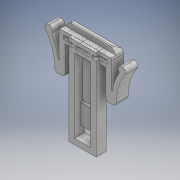
# Autodesk Inventor part: D5MG_Clip
Saved by Autodesk Inventor 2018 (Build 220112000, 112)
## iProperties
Created: 2017-08-14
Part Number: D5MG_Clip
Material: Типовые
Document SubType Name: Modeling
Designer: shawn
Density: 1 g/cm^3
Appearance: По умолчанию
Author: shawn
Autodesk Inventor part; units mm, degrees
ref_plane "YZ Plane" through (0, 0, 0) normal (1, 0, 0) x (0, 1, 0)
ref_plane "XZ Plane" through (0, 0, 0) normal (0, 1, 0) x (-1, 0, 0)
ref_plane "XY Plane" through (0, 0, 0) normal (0, 0, 1) x (1, 0, 0)
sketch "Эскиз1" plane through (0, 0, 0) normal (0, 1, 0) x (-1, 0, 0)
  line L0 (4.8, 15.9) -> (-4.8, 15.9)
  line L1 (-4.8, 15.9) -> (-4.8, -15.9)
  line L2 (-4.8, -15.9) -> (4.8, -15.9)
  line L3 (4.8, -15.9) -> (4.8, 15.9)
  line L4 (4.8, 15.9) -> (-4.8, -15.9) construction
  line L5 (-4.8, 15.9) -> (4.8, -15.9) construction
  line L6 (2.8, -13.9) -> (-2.8, -13.9)
  line L7 (-2.8, -13.9) -> (-2.8, 12.1)
  line L8 (-2.8, 12.1) -> (2.8, 12.1)
  line L9 (2.8, 12.1) -> (2.8, -13.9)
  point P0 (0, 0)
  dimension "d0" = 31.8
  dimension "d1" = 9.6
  dimension "d54" = 2
  dimension "d55" = 2
  dimension "d56" = 2
  dimension "d57" = 3.8
  constraints: 20 end point, 4 parallel, 2 horizontal, 2 midpoint, 2 perpendicular
  measures "d0" distance of L0.end L1.end
  measures "d1" distance of L1.end L2.end
  measures "d54" distance between parallel lines of L3 L9
  measures "d55" distance between parallel lines of L2 L6
  measures "d56" distance between parallel lines of L1 L7
  measures "d57" distance between parallel lines of L0 L8
extrude "Выдавливание1" add sketch "Эскиз1" along normal blind 3.5
ref_plane "РабПлоскость1" through (0, 1, 0) normal (0, -1, 0) x (1, 0, 0)
sketch "Эскиз2" plane through (0, 1, 0) normal (0, -1, 0) x (1, 0, 0)
  line L0 (-4.8, -15.9) -> (-4.8, 15.9) projected
  arc A0 (-13.8048, 12.9671) -> (-14.1893, 13.5232) centre (-28.8, 3.01) ccw
  arc A1 (-13.05, 15.1) -> (-13.8048, 12.9671) centre (-13.05, 13.9) ccw
  line L1 (-4.8, 15.9) -> (4.8, 15.9) projected
  line L2 (-4.8, 12.1) -> (-7.1, 12.1)
  line L3 (-7.1, 12.1) -> (-7.1, 3.1)
  line L4 (-8.3, 1.9) -> (-9.6, 1.9)
  arc A2 (-8.3, 1.9) -> (-7.1, 3.1) centre (-8.3, 3.1) ccw
  arc A3 (-10.8002, 3.1) -> (-9.6, 1.9) centre (-9.6, 3.1002) ccw
  arc A4 (-9.449, 6.1241) -> (-13.3444, 15.0633) centre (-28.8, 3.01) ccw
  arc A5 (-9.449, 6.1241) -> (-9.25, 6.1469) centre (-9.35, 6.14) ccw
  line L5 (0, 0) -> (0, 27.8748) construction
  line L6 (0, 15.8) -> (-9.25, 15.8)
  line L7 (-9.25, 15.8) -> (-9.25, 6.14)
  line L8 (-4.8, 12.1) -> (0, 12.1)
  line L9 (-13.05, 13.9) -> (-12.65, 13.9) construction
  arc A6 (-11.9104, 12.955) -> (-12.65, 15.1) centre (-12.65, 13.9) ccw
  arc A7 (-10.8002, 3.0892) -> (-14.1893, 13.5232) centre (-28.8, 3.01) ccw
  line L10 (-13.05, 15.1) -> (-12.65, 15.1)
  line L11 (4.8, -15.9) -> (4.8, 15.9)
  arc A8 (14.1893, 13.5232) -> (13.8048, 12.9671) centre (28.8, 3.01) ccw
  arc A9 (13.8048, 12.9671) -> (13.05, 15.1) centre (13.05, 13.9) ccw
  line L12 (4.8, 15.9) -> (-4.8, 15.9)
  line L13 (4.8, 12.1) -> (7.1, 12.1)
  line L14 (7.1, 12.1) -> (7.1, 3.1)
  line L15 (8.3, 1.9) -> (9.6, 1.9)
  arc A10 (7.1, 3.1) -> (8.3, 1.9) centre (8.3, 3.1) ccw
  arc A11 (9.6, 1.9) -> (10.8002, 3.1) centre (9.6, 3.1002) ccw
  arc A12 (13.3444, 15.0633) -> (9.449, 6.1241) centre (28.8, 3.01) ccw
  arc A13 (9.25, 6.1469) -> (9.449, 6.1241) centre (9.35, 6.14) ccw
  line L16 (0, 15.8) -> (9.25, 15.8)
  line L17 (9.25, 15.8) -> (9.25, 6.14)
  line L18 (4.8, 12.1) -> (0, 12.1)
  line L19 (13.05, 13.9) -> (12.65, 13.9) construction
  arc A14 (12.65, 15.1) -> (11.9104, 12.955) centre (12.65, 13.9) ccw
  arc A15 (14.1893, 13.5232) -> (10.8002, 3.0892) centre (28.8, 3.01) ccw
  line L20 (13.05, 15.1) -> (12.65, 15.1)
  dimension "d7" = 2.4
  dimension "d13" = 2
  dimension "d14" = 12.89
  dimension "d15" = 24
  dimension "d16" = 8.25
  dimension "d17" = 1.2
  dimension "d19" = 1.3
  dimension "d20" = 2.3
  dimension "d21" = 9
  dimension "d22" = 3.8
  dimension "d23" = 39.2
  dimension "d25" = 9.76
  dimension "d26" = 4.55
  dimension "d27" = 0.1
  dimension "d28" = 4.45
  dimension "d29" = 9.66
  dimension "d30" = 0.4
  dimension "d31" = 2.4
  dimension "d32" = 36
  constraints: 42 point on circle, 38 end point, 29 symmetric about line, 16 centre point, 6 coincident, 6 point on line, 5 tangent, 4 perpendicular, 2 horizontal, 2 vertical, 8 other
  measures "d7" diameter of A1
  measures "d13" distance from line of L9.start L1
  measures "d14" distance from line of L1 A0.centre
  measures "d15" distance from line of L0 A0.centre
  measures "d16" distance from line of L0 L9.start
  measures "d17" radius of A2
  measures "d19" distance of L4.start L4.end
  measures "d20" distance of L2.start L2.end
  measures "d21" distance of L2.end L3.end
  measures "d22" distance between parallel lines of L2 L1
  measures "d23" diameter of A4
  measures "d25" distance from line of L1 A5.centre
  measures "d26" distance from line of L0 A5.centre
  measures "d27" distance between parallel lines of L1 L6
  measures "d28" distance between parallel lines of L0 L7
  measures "d29" distance of L6.end L7.end
  measures "d30" distance of L9.start L9.end
  measures "d31" diameter of A6
  measures "d32" diameter of A7
extrude "Выдавливание2" add sketch "Эскиз2" against normal blind 4.2 contours L2 L3 A2 L4 A3 A7 A0 A1 A4 A5 L7 L6 L0 | L0 L6 L16 L11 L18 L8 | L11 L16 L17 A13 A12 A9 A8 A15 A11 L15 A10 L14 L13 | A4 A1 L10 A6 | A14 L20 A9 A12
sketch "Эскиз3" plane through (-4.8, 0, 15.9) normal (0, 0, 1) x (1, 0, 0)
  line L0 (-2.3, 1) -> (0, 1) projected
  line L1 (9.6, 3.5) -> (0, 3.5) projected
  line L2 (0, 1) -> (9.6, 1)
  line L3 (9.6, 1) -> (9.6, 3.5)
  line L4 (9.6, 3.5) -> (0, 3.5)
  line L5 (0, 3.5) -> (0, 1)
  point P0 (4.8, 0)
  constraints: 8 end point, 2 parallel, 1 horizontal, 1 perpendicular
extrude "Выдавливание3" cut sketch "Эскиз3" against normal up to surface (0.1 mm away)
sketch "Эскиз4" plane through (0, 5.2, 0) normal (0, 1, 0) x (1, 0, 0)
  line L0 (-2.35, -14.6) -> (2.35, -14.6)
  line L1 (2.35, -14.6) -> (2.35, -13.4)
  line L2 (2.35, -13.4) -> (-2.35, -13.4)
  line L3 (-2.35, -13.4) -> (-2.35, -14.6)
  line L4 (-2.35, -14.6) -> (2.35, -13.4) construction
  line L5 (2.35, -14.6) -> (-2.35, -13.4) construction
  line L6 (4.8, -15.9) -> (-4.8, -15.9) projected
  line L7 (0, 0) -> (0, -15.9) construction
  line L8 (-3.35, -14.6) -> (-7.7, -14.6)
  line L9 (-7.7, -14.6) -> (-7.7, -13.4)
  line L10 (-7.7, -13.4) -> (-3.35, -13.4)
  line L11 (-3.35, -13.4) -> (-3.35, -14.6)
  line L12 (3.35, -14.6) -> (7.7, -14.6)
  line L13 (7.7, -14.6) -> (7.7, -13.4)
  line L14 (7.7, -13.4) -> (3.35, -13.4)
  line L15 (3.35, -13.4) -> (3.35, -14.6)
  point P0 (0, -14)
  point P1 (0, -14)
  dimension "d37" = 1.2
  dimension "d38" = 1.3
  dimension "d39" = 4.7
  dimension "d40" = 4.35
  dimension "d41" = 1
  constraints: 30 end point, 4 midpoint, 4 parallel, 4 symmetric about line, 2 collinear, 2 horizontal, 2 perpendicular, 1 point on line
  measures "d37" distance of L0.end L1.end
  measures "d38" distance between parallel lines of L0 L6
  measures "d39" distance of L0.start L0.end
  measures "d40" distance of L9.end L10.end
  measures "d41" distance between parallel lines of L3 L11
extrude "Выдавливание4" cut sketch "Эскиз4" against normal through all
sketch "Эскиз5" plane through (-9.25, 5.2, 15.8) normal (0, 0, 1) x (1, 0, 0)
  line L0 (0, 0) -> (18.5, 0) projected
  line L1 (0, 0) -> (18.5, 0)
  line L2 (18.5, 0) -> (18.5, -2.4)
  line L3 (18.5, -2.4) -> (0, -2.4)
  line L4 (0, -2.4) -> (0, 0)
  line L5 (18.5, -4.2) -> (18.5, 0) projected
  point P0 (9.25, -5.2)
  dimension "d44" = 2.4
  constraints: 8 end point, 2 parallel, 1 collinear, 1 horizontal, 1 perpendicular
  measures "d44" distance of L1.end L2.end
extrude "Выдавливание5" add sketch "Эскиз5" along normal blind 1.8
chamfer "Фаска1" distance 1.9 distance2 1.1 1 edges at (0, 5.2, 17.6) measured on face at (0, 4.7, 17.6)
chamfer "Фаска2" distance 2 angle 45 2 edges at (-9.25, 3.05, 17.6) (9.25, 3.05, 17.6)
fillet "Сопряжение1" radius 0.75 4 edges at (-9.25, 3.1, 15.6) (-7.25, 3.05, 17.6) (7.25, 3.05, 17.6) (9.25, 3.1, 15.6)
sketch "Эскиз6" plane through (0, 3.5, 0) normal (0, 1, 0) x (1, 0, 0)
  line L0 (-2.8, -12.1) -> (-2.8, 13.9) projected
  line L1 (2.8, 13.9) -> (2.8, -12.1) projected
  line L2 (-2.8, 10.9) -> (2.8, 10.9)
  line L3 (2.8, 10.9) -> (2.8, 3.9)
  line L4 (2.8, 3.9) -> (-2.8, 3.9)
  line L5 (-2.8, 3.9) -> (-2.8, 10.9)
  line L6 (4.8, 15.9) -> (-4.8, 15.9) projected
  line L7 (0, 0) -> (0, -12.1) construction
  line L8 (-2.8, -12.1) -> (2.8, -12.1) construction
  line L9 (-2, -12.1) -> (2, -12.1)
  line L10 (2, -12.1) -> (2, 2.9)
  line L11 (2, 2.9) -> (-2, 2.9)
  line L12 (-2, 2.9) -> (-2, -12.1)
  line L13 (-2, -12.1) -> (2, 2.9) construction
  line L14 (2, -12.1) -> (-2, 2.9) construction
  line L15 (7.1, -12.1) -> (-7.1, -12.1) projected
  point P0 (0, -4.6)
  dimension "d58" = 5
  dimension "d59" = 7
  dimension "d60" = 13
  dimension "d61" = 4
  constraints: 22 end point, 4 parallel, 3 midpoint, 3 point on line, 2 horizontal, 2 perpendicular, 1 collinear
  measures "d58" distance between parallel lines of L6 L2
  measures "d59" distance between parallel lines of L2 L4
  measures "d60" distance between parallel lines of L6 L11
  measures "d61" distance of L10.end L11.end
extrude "Выдавливание6" add sketch "Эскиз6" against normal blind 1.5 contours L0 L2 L1 L4 | L12 L11 L10 L9
sketch "Эскиз7" plane through (0, 3.5, 0) normal (0, 1, 0) x (1, 0, 0)
  line L0 (-2, 2.9) -> (-2, -12.1) projected
  line L1 (2, -12.1) -> (2, 2.9) projected
  line L2 (-2, 2.9) -> (2, 2.9)
  line L3 (2, 2.9) -> (2, -2.0018)
  line L4 (2, -2.0018) -> (-2, -2.0018)
  line L5 (-2, -2.0018) -> (-2, 2.9)
  point P0 (0, 0)
  constraints: 8 end point, 2 parallel, 1 horizontal, 1 perpendicular, 1 point on line
extrude "Выдавливание7" add sketch "Эскиз7" along normal blind 1.7
chamfer "Фаска3" distance 3.7 distance2 1.7 1 edges at (0, 5.2, -2.9) measured on face at (0, 5.2, -2.4)
sketch "Эскиз8" plane through (0, 3.5, 0) normal (0, 1, 0) x (1, 0, 0)
  line L0 (-2.8, -12.1) -> (-2.8, 3.9) projected
  line L1 (-4.8, -12.1) -> (-2.8, -12.1)
  line L2 (-2.8, -12.1) -> (-2.8, -10.357)
  line L3 (-2.8, -10.357) -> (-4.8, -10.357)
  line L4 (-4.8, -10.357) -> (-4.8, -12.1)
  line L5 (2.8, 3.9) -> (2.8, -12.1) projected
  line L6 (2.8, -12.1) -> (4.8, -12.1)
  line L7 (4.8, -12.1) -> (4.8, -10.357)
  line L8 (4.8, -10.357) -> (2.8, -10.357)
  line L9 (2.8, -10.357) -> (2.8, -12.1)
  line L10 (4.8, -12.1) -> (4.8, 15.9) projected
  point P0 (0, 0)
  constraints: 16 end point, 4 parallel, 2 horizontal, 2 perpendicular, 2 point on line, 1 collinear
extrude "Выдавливание8" add sketch "Эскиз8" along normal up to surface (1.7 mm away)
